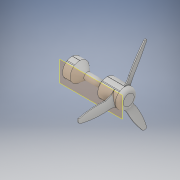
# Autodesk Inventor part: fixed prop
Saved by Autodesk Inventor 2019 (Build 230136000, 136)
## iProperties
Created: 2020-03-27
Part Number: fixed prop
Material: Generic
Document SubType Name: Modeling
Designer: q
Density: 1 g/cm^3
Appearance: Default
Author: q
Autodesk Inventor part; units mm, degrees
ref_plane "YZ Plane" through (0, 0, 0) normal (1, 0, 0) x (0, 1, 0)
ref_plane "XZ Plane" through (0, 0, 0) normal (0, 1, 0) x (-1, 0, 0)
ref_plane "XY Plane" through (0, 0, 0) normal (0, 0, 1) x (1, 0, 0)
sketch "Sketch1" plane through (0, 0, 0) normal (1, 0, 0) x (0, 1, 0)
  line L0 (0, 0) -> (125, 0)
  line L1 (0, 0) -> (-125, 0)
  line L2 (0, 0) -> (0, -125)
  arc A0 (-125, 0) -> (125, 0) centre (0, 0) ccw
  dimension "d0" = 125
  dimension "d1" = 125
  dimension "d2" = 125
  constraints: 6 end point, 3 point on circle, 2 horizontal, 1 centre point, 1 vertical
  measures "d0" distance of L0.start L0.end
  measures "d1" distance of L0.start L1.end
  measures "d2" distance of L0.start L2.end
extrude "Extrusion1" add sketch "Sketch1" along normal blind 750
sketch "Sketch2" plane through (0, -125, 0) normal (0, 0, 1) x (1, 0, 0)
  line L0 (0, 125) -> (67.1182, 125)
  line L1 (0, 0) -> (0, 250) projected
  line L2 (0, 0) -> (750, 0) projected
  line L3 (0, 0) -> (100, 0)
  line L4 (100, 0) -> (200, 0)
  line L5 (100, 0) -> (200, 80.3651)
  line L6 (200, 80.3651) -> (400, 80.3651)
  line L7 (400, 80.3651) -> (464.5856, 0)
  line L8 (464.5856, 0) -> (634.3266, 0)
  line L9 (750, 0) -> (750, 250) projected
  line L10 (634.3266, 0) -> (750, 0)
  line L11 (750, 0) -> (750, 125)
  line L12 (750, 125) -> (67.1182, 125)
  dimension "d5" = 100
  dimension "d6" = 100
  dimension "d7" = 200
  constraints: 20 end point, 4 point on line, 3 horizontal, 1 midpoint, 1 perpendicular
  measures "d5" distance of L1.start L3.end
  measures "d6" distance of L3.end L4.end
  measures "d7" distance of L5.end L6.end
revolve "Revolution1" cut sketch "Sketch2" angle 360 about axis through (0, 0, 0) along (1, 0, 0) contours L5 L6 L7 L2
ref_plane "Work Plane1" through (0, -125, 125) normal (0, 0, 1) x (1, 0, 0)
sketch "Sketch3" plane through (0, -125, 125) normal (0, 0, 1) x (1, 0, 0)
  arc A0 (691.7068, 67.7419) -> (628.6973, 233.1419) centre (365.4488, 38.155) ccw
  arc A1 (679.8925, 67.7419) -> (691.7068, 67.7419) centre (685.7996, 72.1574) ccw
  arc A2 (679.8925, 67.7419) -> (628.6973, 233.1419) centre (-45.6941, -66.2213) ccw
  point P0 (0, 125)
  constraints: 6 point on circle, 3 centre point
sketch "Sketch4" plane through (0, -125, 0) normal (0, 0, 1) x (1, 0, 0)
  line L0 (0, 250) -> (0, 0) projected
  line L1 (0, 250) -> (0, 0)
  line L2 (0, 0) -> (100, 0) projected
  line L3 (0, 0) -> (100, 0)
  line L4 (100, 0) -> (200, 80.3651) projected
  line L5 (100, 0) -> (200, 80.3651)
  line L6 (400, 169.6349) -> (400, 80.3651) projected
  line L7 (200, 80.3651) -> (400, 80.3651)
  line L8 (400, 80.3651) -> (464.5856, 0) projected
  line L9 (400, 80.3651) -> (464.5856, 0)
  line L10 (464.5856, 0) -> (750, 0) projected
  line L11 (464.5856, 0) -> (750, 0)
  line L12 (750, 0) -> (750, 125)
  line L13 (750, 250) -> (750, 0) projected
  line L14 (0, 125) -> (750, 125)
  constraints: 16 end point, 4 collinear, 1 midpoint, 1 parallel, 1 perpendicular, 1 vertical
revolve "Revolution2" add sketch "Sketch4" angle 360 about axis through (0, 0, 0) along (1, 0, 0)
extrude "Extrusion2" add sketch "Sketch3" against normal up to next
sketch "Sketch5" plane through (0, -125, 125) normal (0, 0, 1) x (1, 0, 0)
  arc A0 (691.7068, 67.7419) -> (681.3247, 125) centre (365.4488, 38.155) ccw projected
  arc A1 (681.3247, 125) -> (628.6973, 233.1419) centre (365.4488, 38.155) ccw projected
  arc A2 (691.7068, 67.7419) -> (628.6973, 233.1419) centre (365.4488, 38.155) ccw
  arc A3 (679.8925, 67.7419) -> (691.7068, 67.7419) centre (685.7996, 72.1574) ccw projected
  arc A4 (679.8925, 67.7419) -> (691.7068, 67.7419) centre (685.7996, 72.1574) ccw
  arc A5 (679.8925, 67.7419) -> (666.9464, 125) centre (-45.6941, -66.2213) ccw projected
  arc A6 (666.9464, 125) -> (628.6973, 233.1419) centre (-45.6941, -66.2213) ccw projected
  arc A7 (679.8925, 67.7419) -> (628.6973, 233.1419) centre (-45.6941, -66.2213) ccw
  point P0 (0, 125)
  constraints: 8 point on circle, 3 centre point
extrude "Extrusion3" add sketch "Sketch5" along normal blind 500
pattern_circular "Circular Pattern1" count 3 over 360 about axis through (0, 0, 0) along (1, 0, 0) of "Extrusion2"
sketch "Sketch6" plane through (685.7996, -81.8319, -108.263) normal (0, -0.8660254, -0.5) x (1, 0, 0)
  arc A0 (5.9071, -4.4155) -> (-4.4749, 52.8426) centre (-320.3508, -34.0024) ccw projected
  arc A1 (-18.8532, 52.8426) -> (-57.1024, 160.9845) centre (-731.4937, -138.3787) ccw projected
  arc A2 (-4.4749, 52.8426) -> (-57.1024, 160.9845) centre (-320.3508, -34.0024) ccw projected
  arc A3 (5.9071, -4.4155) -> (-57.1024, 160.9845) centre (-320.3508, -34.0024) ccw
  arc A4 (-5.9071, -4.4155) -> (5.9071, -4.4155) centre (0, 0) ccw projected
  arc A5 (-5.9071, -4.4155) -> (5.9071, -4.4155) centre (0, 0) ccw
  arc A6 (-5.9071, -4.4155) -> (-18.8532, 52.8426) centre (-731.4937, -138.3787) ccw projected
  arc A7 (-5.9071, -4.4155) -> (-57.1024, 160.9845) centre (-731.4937, -138.3787) ccw
  point P0 (-685.7996, 52.8426)
  constraints: 8 point on circle, 3 centre point
extrude "Extrusion4" add sketch "Sketch6" along normal blind 500
sketch "Sketch7" plane through (685.7996, 134.6745, -16.737) normal (0, 0.8660254, -0.5) x (1, 0, 0)
  arc A0 (5.9071, -4.4155) -> (-4.4749, 52.8426) centre (-320.3508, -34.0024) ccw projected
  arc A1 (-18.8532, 52.8426) -> (-57.1024, 160.9845) centre (-731.4937, -138.3787) ccw projected
  arc A2 (5.9071, -4.4155) -> (-57.1024, 160.9845) centre (-320.3508, -34.0024) ccw
  arc A3 (-5.9071, -4.4155) -> (-18.8532, 52.8426) centre (-731.4937, -138.3787) ccw projected
  arc A4 (-5.9071, -4.4155) -> (5.9071, -4.4155) centre (0, 0) ccw
  arc A5 (-5.9071, -4.4155) -> (-57.1024, 160.9845) centre (-731.4937, -138.3787) ccw
  point P0 (-685.7996, 52.8426)
  constraints: 7 point on circle, 3 centre point
extrude "Extrusion5" add sketch "Sketch7" along normal blind 500
sketch "Sketch8" plane through (750, 0, 0) normal (1, 0, 0) x (0, 0, -1)
  circle A0 centre (0, 0) radius 125 projected
  circle A1 centre (0, 0) radius 625
  line L0 (362.0869, -512.6368) -> (218.8464, -595.3368) projected
  constraints: 1 centre point, 1 coincident, 1 tangent
extrude "Extrusion6" cut sketch "Sketch8" against normal blind 856 contours A0 | A1 keep common part
fillet "Fillet1" radius 4.75 5 edges at (649.6069, 511.2523, -359.5081) (673.9752, 554.9247, -287.5476) (659.1047, 509.7183, -361.6798) (687.7613, 554.834, -287.7224) (685.7996, 568.8565, -258.8962)
pattern_circular "Circular Pattern2" count 3 over 360 about axis through (0, 0, 0) along (1, 0, 0) of "Fillet1"
fillet "Fillet2" radius 53.25 1 edges at (750, 125, 0)
sketch "Sketch9" plane through (750, 0, 0) normal (1, 0, 0) x (0, 0, -1)
  circle A0 centre (0, 0) radius 125 projected
  arc A1 (-219.7991, 51.9836) -> (-62.6924, 108.1419) centre (-256.8968, 403.6045) ccw
  arc A2 (-110.7523, -57.9562) -> (-219.7991, -44.6484) centre (-182.9956, -196.5036) ccw
  arc A3 (-579.1494, -14.4509) -> (-219.7991, -44.6484) centre (-287.7435, 1300.0466) ccw
  arc A4 (-219.7991, 51.9836) -> (-579.1494, 31.8519) centre (-315.9278, -1449.386) ccw
  line L0 (-62.6924, 108.1419) -> (-610.4055, 108.1419) projected
  arc A5 (-62.6924, 108.1419) -> (-110.7523, -57.9562) centre (2.2792, -0.6595) ccw
  arc A6 (-579.1494, 31.8519) -> (-579.1494, -14.4509) centre (-565.2121, 8.7005) ccw
  arc A7 (64.8804, -216.3434) -> (261.9901, -517.484) centre (1413.169, 451.0915) ccw
  arc A8 (64.8804, -216.3434) -> (-62.3074, -108.3641) centre (-221.0833, -424.2814) ccw
  arc A9 (-62.3074, -108.3641) -> (105.5677, -66.9363) centre (-0.5685, 2.3036) ccw
  arc A10 (105.5677, -66.9363) -> (148.5662, -168.0274) centre (261.6749, -60.2271) ccw
  arc A11 (302.0896, -494.3326) -> (148.5662, -168.0274) centre (-982.0017, -899.2165) ccw
  arc A12 (261.9901, -517.484) -> (302.0896, -494.3326) centre (275.0712, -493.8383) ccw
  arc A13 (154.9186, 164.3598) -> (317.1593, 485.6321) centre (-1097.2412, 998.2945) ccw
  arc A14 (154.9186, 164.3598) -> (124.9998, 0.2223) centre (477.9801, 20.6769) ccw
  arc A15 (124.9998, 0.2223) -> (5.1847, 124.8924) centre (-1.7108, -1.6441) ccw
  arc A16 (5.1847, 124.8924) -> (71.2329, 212.6758) centre (-78.6793, 256.7307) ccw
  arc A17 (277.0598, 508.7835) -> (71.2329, 212.6758) centre (1269.7451, -400.8302) ccw
  arc A18 (317.1593, 485.6321) -> (277.0598, 508.7835) centre (290.1409, 485.1378) ccw
  line L1 (-62.6924, 108.1419) -> (-610.4055, 108.1419)
  line L2 (-646.2627, 108.1419) -> (-657.1252, -85.2428)
  line L3 (-657.1252, -85.2428) -> (-619.1064, -66.9363)
  line L4 (-619.1064, -66.9363) -> (-110.7523, -57.9562)
  line L5 (-610.4055, 108.1419) -> (-646.2627, 108.1419)
  dimension "d31" = 360
  constraints: 37 point on circle, 18 centre point, 10 end point, 2 collinear, 1 point on line, 55 other
extrude "Extrusion7" cut sketch "Sketch9" against normal blind 856 contours A5 A1 A0 | A0 A1 A4 A6 A3 A2 L4 L3 L2 L5 L0 | A1 A5 picked at (-68.4274, 104.5344)
pattern_circular "Circular Pattern3" count 3 over 360 about axis through (0, 0, 0) along (1, 0, 0) of "Extrusion7"
sketch "Sketch10" plane through (750, 0, 0) normal (1, 0, 0) x (0, 0, -1)
  line L0 (171.5352, -176.6724) -> (105.5677, -66.9363) projected
  line L1 (105.5677, -66.9363) -> (106.9196, -64.7549)
  line L2 (171.5352, -176.6724) -> (106.9196, -64.7549) projected
  line L3 (106.9196, -64.7549) -> (174.2794, -175.1388)
  line L4 (174.2794, -175.1388) -> (169.9055, -179.8492)
  line L5 (169.9055, -179.8492) -> (105.5677, -66.9363)
  line L6 (5.1847, 124.8924) -> (2.6196, 124.9725)
  line L7 (2.6196, 124.9725) -> (64.535, 238.4998)
  line L8 (64.535, 238.4998) -> (70.8012, 237.0671)
  line L9 (70.8012, 237.0671) -> (5.1847, 124.8924)
  line L10 (-110.7523, -57.9562) -> (-109.5392, -60.2176)
  line L11 (-109.5392, -60.2176) -> (-238.8144, -63.361)
  line L12 (-238.8144, -63.361) -> (-240.7067, -57.2179)
  line L13 (-240.7067, -57.2179) -> (-110.7523, -57.9562)
  point P0 (0, 0)
  dimension "d40" = 360
  constraints: 24 end point, 1 point on line, 25 other
extrude "Extrusion8" cut sketch "Sketch10" against normal blind 856
body "Solid1"
